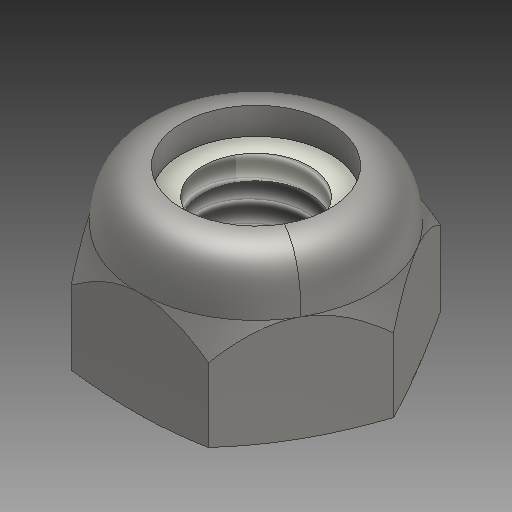
# Autodesk Inventor part: HexNut_0.875inch
Saved by Autodesk Inventor 2019 (Build 230136000, 136)
## iProperties
Created: 2020-12-09
Part Number: HexNut_0.875inch
Material: Generic
Document SubType Name: Modeling
Designer: Anass Hamdi
Density: 1 g/cm^3
Appearance: Default
Mass: 0.275597 g
Surface Area: 3.81681 cm^2
Volume: 0.275597 cm^3
Author: Anass Hamdi
Autodesk Inventor part; units mm, degrees
sketch "Sketch1" plane through (0, 0, 0) normal (0, 0, 1) x (1, 0, 0)
  line L0 (0, 5.055) -> (4.3778, 2.5275)
  line L1 (4.3778, 2.5275) -> (4.3778, -2.5275)
  line L2 (4.3778, -2.5275) -> (0, -5.055)
  line L3 (0, -5.055) -> (-4.3778, -2.5275)
  line L4 (-4.3778, -2.5275) -> (-4.3778, 2.5275)
  line L5 (-4.3778, 2.5275) -> (0, 5.055)
  point P0 (0, 0)
  point P1 (0, 0)
  dimension "d1" = 10.11
  dimension "d20" = 8.7555
  constraints: 12 end point, 1 coincident, 13 other
  measures "d1" distance of L2.end L0.start
  measures "d20" distance between parallel lines of L1 L4
extrude "Extrusion1" add sketch "Sketch1" along normal blind 3.93
ref_plane "Work Plane1" through (0, 0, 2.93) normal (0, 0, 1) x (1, 0, 0)
ref_plane "Work Plane2" through (0, 0, 0.2) normal (0, 0, -1) x (-1, 0, 0)
sketch "Sketch9" plane through (0, 0, 2.93) normal (0, 0, 1) x (1, 0, 0)
  line L0 (-5.1098, 2.8214) -> (-2.6107, 4.3287)
  line L1 (-5.0541, -0.0966) -> (-5.1098, 2.8214)
  arc A0 (-2.6107, 4.3287) -> (-5.0541, -0.0966) centre (0, 0) ccw
  point P0 (-4.3778, 2.5275)
  constraints: 4 end point, 3 point on circle, 1 centre point, 1 tangent
sketch "Sketch10" plane through (0, 0, 3.93) normal (0, 0, 1) x (1, 0, 0)
  line L0 (-4.3778, 0) -> (-4.3778, 2.5275)
  line L1 (-4.3778, 2.5275) -> (-2.1889, 3.7912)
  arc A0 (-2.1889, 3.7912) -> (-4.3778, 0) centre (0, 0) ccw
  constraints: 4 end point, 2 point on circle, 1 centre point
loft "Loft4" cut profiles "Sketch9", "Sketch10"
pattern_circular "Circular Pattern3" count 6 over 360 about axis through (0, 0, -10) along (0, 0, 1) of "Loft4"
sketch "Sketch11" plane through (0, 0, 0) normal (0, 0, -1) x (-1, 0, 0)
  line L0 (-4.3778, 0) -> (-4.3778, 2.5275)
  line L1 (-4.3778, 2.5275) -> (-2.1889, 3.7912)
  arc A0 (-2.1889, 3.7912) -> (-4.3778, 0) centre (0, 0) ccw
  constraints: 4 end point, 2 point on circle, 1 centre point
sketch "Sketch12" plane through (0, 0, 0.2) normal (0, 0, -1) x (-1, 0, 0)
  line L0 (-5.1098, 2.8214) -> (-2.6107, 4.3287)
  line L1 (-5.0541, -0.0966) -> (-5.1098, 2.8214)
  arc A0 (-2.6107, 4.3287) -> (-5.0541, -0.0966) centre (0, 0) ccw
  point P0 (-4.3778, 2.5275)
  constraints: 4 end point, 3 point on circle, 1 centre point, 1 tangent
loft "Loft5" cut profiles "Sketch11", "Sketch12"
pattern_circular "Circular Pattern4" count 6 over 360 about axis through (0, 0, -10) along (0, 0, 1) of "Loft5"
sketch "Sketch17" plane through (0, 0, 0) normal (1, 0, 0) x (0, 1, 0)
  line L0 (-4.3778, 3.93) -> (4.3778, 3.93) projected
  line L1 (5.055, 2.93) -> (5.055, 0.2) projected
  line L2 (4.3778, 0) -> (-4.3778, 0) projected
  line L3 (-5.055, 0.2) -> (-5.055, 2.93) projected
  line L4 (0, 3.93) -> (0, 5.82)
  line L5 (0, 5.82) -> (-2.754, 5.82)
  line L6 (-2.754, 5.82) -> (-2.754, 3.93)
  line L7 (0, 3.93) -> (-2.754, 3.93)
  point P0 (0, 0)
  dimension "d53" = 1.89
  dimension "d54" = 2.754
  constraints: 8 end point, 2 perpendicular, 1 collinear, 1 midpoint, 1 point on line, 1 vertical, 4 other
  measures "d53" distance of L4.start L4.end
  measures "d54" distance of L4.end L5.end
revolve "Revolution2" add sketch "Sketch17" angle 360 about axis through (0, 0, 3.93) along (0, 0, 1)
ref_plane "Work Plane5" through (4.3778, 0, 3.93) normal (0, 0, 1) x (1, 0, 0)
split body "Split1" result two bodies by plane through (4.3778, 0, 3.93) normal (0, 0, 1) first body at (-0.1814, -2.2467, 5.19)
sketch "Sketch21" plane through (0, 0, 0) normal (0, 1, 0) x (-1, 0, 0)
  line L0 (-2.754, 3.93) -> (-2.754, 5.82)
  line L1 (-4.3778, 3.93) -> (-4.3778, 5.82) construction
  line L2 (-4.3778, 5.82) -> (-2.754, 5.82) construction
  spline S0 degree 2 poles (-4.3778, 3.93) (-4.3778, 5.82) (-2.754, 5.82) knots 1 1 1 2 2 2
  line L3 (-4.3778, 3.93) -> (-2.754, 3.93)
  line L4 (-2.754, 5.82) -> (-2.754, 3.93)
  line L5 (-2.754, 3.93) -> (-2.754, 5.82) projected
  line L6 (0, -1.2519) -> (0, 7.504) projected
  point P0 (0, 0)
  constraints: 6 end point, 1 collinear, 3 other
revolve "Revolution3" add sketch "Sketch21" angle 360 about axis through (0, 0, -10) along (0, 0, 1) bodies 3
sketch "Sketch22" plane through (0, 0, 5.82) normal (0, 0, 1) x (1, 0, 0)
  circle A0 centre (0, 0) radius 2.754
  constraints: 1 centre point, 1 coincident
extrude "Extrusion3" cut sketch "Sketch22" against normal blind 1 bodies 2
sketch "Sketch23" plane through (0, 0, 4.82) normal (0, 0, 1) x (1, 0, 0)
  point P0 (0, 0)
  point P1 (0, 0)
  constraints: 1 coincident
hole "Hole2" at (0, 0, 4.82) direction (0, 0, -1) diameter 3.962 depth 6 bodies 2 thread size "10-32 UNF" class "2B" standard "ANSI Unified Screw Threads"
sketch "Sketch24" plane through (0, 0, 3.93) normal (0, 0, 1) x (1, 0, 0)
  point P0 (0, 0)
  point P1 (0, 0)
  constraints: 1 coincident
hole "Hole3" at (0, 0, 3.93) direction (0, 0, -1) diameter 3.962 depth 4 bodies 3 thread size "10-32 UNF" class "2B" standard "ANSI Unified Screw Threads"
chamfer "Chamfer2" distance 0.3 angle 45 1 edges at (0, 1.981, 0)
body "Solid2"
body "Solid3"
